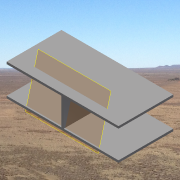
# Autodesk Inventor part: 2p1rim1
Saved by Autodesk Inventor 2014 SP1 (Build 180222100, 222)
## iProperties
Company: HERA Project
Created: 2013-12-03
Part Number: 2p1rim1
Material: Steel, Galvanized
Document SubType Name: Modeling
Designer: David DeBoer
Mass: 492.101 g
Surface Area: 430.611 cm^2
Volume: 62.688 cm^3
Density: 7.85 g/cm^3
Description: end horizontal rim holder 1
Appearance: Galvanized
d2: 0.120 in
d17: 0.120 in
d18: 3.000 in
d19: 0.00 deg
d20: 15.00 deg
d21: -0.500 in
d22: 1.000 in
d23: 0.00 deg
d24: 0.050 in
d25: 0.050 in
d26: 0.005 in
d27: 0.050 in
d28: 0.170 in
d29: 0.00 deg
d30: 0.00 deg
Author: David DeBoer
Autodesk Inventor part; units mm, degrees
ref_plane "YZ Plane" through (0, 0, 0) normal (1, 0, 0) x (0, 1, 0)
ref_plane "XZ Plane" through (0, 0, 0) normal (0, 1, 0) x (-1, 0, 0)
ref_plane "XY Plane" through (0, 0, 0) normal (0, 0, 1) x (1, 0, 0)
sketch "Sketch1" plane through (0, 0, 0) normal (0, 0, 1) x (1, 0, 0)
  line L0 (45.974, 38.1) -> (45.974, 0)
  line L1 (49.022, 38.1) -> (49.022, 0)
  line L2 (49.022, 19.05) -> (99.822, 19.05) construction
  line L3 (45.974, 0) -> (-30.226, 0)
  line L4 (-30.226, 0) -> (-30.226, -3.048)
  line L5 (-30.226, -3.048) -> (125.222, -3.048)
  line L6 (125.222, -3.048) -> (125.222, 0)
  line L7 (125.222, 0) -> (49.022, 0)
  line L8 (45.974, 38.1) -> (-30.226, 38.1)
  line L9 (-30.226, 38.1) -> (-30.226, 41.148)
  line L10 (-30.226, 41.148) -> (125.222, 41.148)
  line L11 (125.222, 41.148) -> (125.222, 38.1)
  line L12 (125.222, 38.1) -> (49.022, 38.1)
  dimension "d17" = 3.048
  dimension "d60" = 50.8
  dimension "d61" = 76.2
  dimension "d62" = 3.048
  dimension "d63" = 90
  dimension "d64" = 155.448
  constraints: 26 end point, 4 parallel, 4 symmetric about line, 2 perpendicular, 2 point on line, 1 midpoint
  measures "d17" distance between parallel lines of L1 L0
  measures "d60" distance of L2.start L2.end
  measures "d61" distance of L0.end L3.end
  measures "d62" distance of L3.end L4.end
  measures "d63" angle of L4 L3
  measures "d64" distance of L4.end L5.end
extrude "Extrusion6" add sketch "Sketch1" along normal blind 76.2
ref_plane "Work Plane4" through (91.948, 37.861, 63.9327) normal (0, 0.258819, 0.9659258) x (-1, 0, 0)
ref_plane "Work Plane3" through (91.948, 41.148, 76.2) normal (0, 0.258819, 0.9659258) x (-1, 0, 0)
sketch "Sketch6" plane through (91.948, 37.861, 63.9327) normal (0, 0.258819, 0.9659258) x (-1, 0, 0)
  line L0 (-2.4638, -7.3313) -> (94.6916, -7.3313)
  line L1 (94.6916, -7.3313) -> (94.6916, 43.8286)
  line L2 (94.6916, 43.8286) -> (-2.4638, 43.8286)
  line L3 (-2.4638, 43.8286) -> (-2.4638, -7.3313)
  point P0 (91.948, 20.0239)
  constraints: 8 end point, 2 parallel, 1 horizontal, 1 perpendicular
extrude "Extrusion7" [suppressed]
sketch "Sketch7" plane through (45.974, 0, 0) normal (-1, 0, 0) x (0, 0, 1)
  line L0 (0, 38.1) -> (76.2, 38.1) projected
  line L1 (62.4717, 38.1) -> (63.7417, 38.1)
  line L2 (63.7417, 38.1) -> (63.7417, 36.83)
  line L3 (63.7417, 36.83) -> (62.4717, 36.83)
  line L4 (62.4717, 36.83) -> (62.4717, 38.1)
  point P0 (63.8687, 38.1)
  dimension "d24" = 1.27
  dimension "d25" = 1.27
  dimension "d26" = 0.127
  constraints: 8 end point, 2 parallel, 1 horizontal, 1 perpendicular, 1 point on line
  measures "d24" distance of L2.end L3.end
  measures "d25" distance of L1.end L2.end
  measures "d26" distance of point (63.869, 38.1) L1.end
extrude "Extrusion8" add sketch "Sketch7" along normal blind 1.27 and the other way blind 4.318
body "Solid2"
